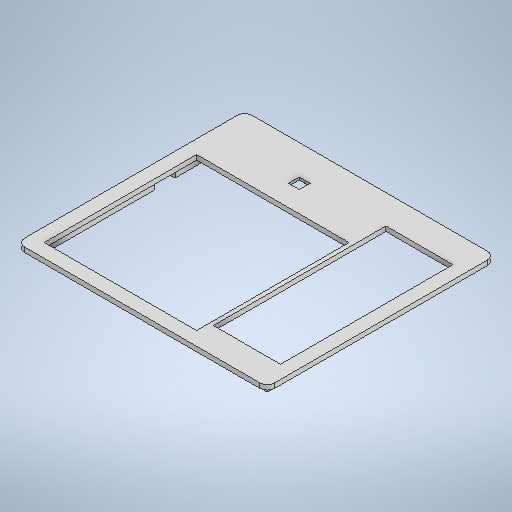
# Autodesk Inventor part: EnclosureLid
Saved by Autodesk Inventor 2025.2 (Build 292293000, 293)
## iProperties
Created: 2025-04-29
Part Number: EnclosureLid
Material: Generic
Document SubType Name: Modeling
Designer: mathe
Density: 1 g/cm^3
Appearance: Default
Author: mathe
Autodesk Inventor part; units mm, degrees
ref_plane "YZ Plane" through (0, 0, 0) normal (1, 0, 0) x (0, 1, 0)
ref_plane "XZ Plane" through (0, 0, 0) normal (0, 1, 0) x (-1, 0, 0)
ref_plane "XY Plane" through (0, 0, 0) normal (0, 0, 1) x (1, 0, 0)
sketch "Sketch1" plane through (0, 0, 0) normal (0, 1, 0) x (-1, 0, 0)
  circle A0 centre (-103.3712, -13.8328) radius 2.5
  circle A1 centre (-103.3712, -93.8328) radius 2.5
  circle A2 centre (-78.3712, -13.8328) radius 2.5
  circle A3 centre (-78.3712, -93.8328) radius 2.5
  line L0 (-8.8712, -9.8328) -> (-107.3712, -9.8328)
  line L1 (-107.3712, -9.8328) -> (-107.3712, -98.8828)
  line L2 (-107.3712, -98.8828) -> (-8.8712, -98.8828)
  line L3 (-8.8712, -98.8828) -> (-8.8712, -69.8328)
  line L4 (-5.8712, -69.8328) -> (-8.8712, -69.8328)
  line L5 (-5.8712, -57.8328) -> (-5.8712, -69.8328)
  line L6 (-5.8712, -57.8328) -> (-8.8712, -57.8328)
  line L7 (-8.8712, -57.8328) -> (-8.8712, -9.8328)
  line L8 (-8.8712, -57.8328) -> (-6.8712, -57.8328)
  line L9 (-6.8712, -57.8328) -> (-6.8712, -69.8328)
  line L10 (-6.8712, -69.8328) -> (-8.8712, -69.8328)
  line L11 (-8.8712, -69.8328) -> (-8.8712, -98.8828)
  line L12 (-8.8712, -98.8828) -> (-107.3712, -98.8828)
  line L13 (-107.3712, -98.8828) -> (-107.3712, -9.8328)
  line L14 (-107.3712, -9.8328) -> (-8.8712, -9.8328)
  line L15 (-8.8712, -9.8328) -> (-8.8712, -57.8328)
  line L16 (-5.8712, -6.8328) -> (-110.3712, -6.8328)
  line L17 (-110.3712, -6.8328) -> (-110.3712, -101.8828)
  line L18 (-110.3712, -101.8828) -> (-5.8712, -101.8828)
  line L19 (-5.8712, -101.8828) -> (-5.8712, -6.8328)
  line L20 (-103.3712, -93.8328) -> (-78.3712, -93.8328) construction
  line L21 (-78.3712, -93.8328) -> (-78.3712, -13.8328) construction
  line L22 (-78.3712, -13.8328) -> (-103.3712, -13.8328) construction
  line L23 (-103.3712, -13.8328) -> (-103.3712, -93.8328) construction
  line L24 (-90.8712, -93.8328) -> (-90.8712, -13.8328) construction
  line L25 (-103.3712, -53.8328) -> (-78.3712, -53.8328) construction
  line L26 (-76.8712, -89.8328) -> (-104.8712, -89.8328)
  line L27 (-104.8712, -89.8328) -> (-104.8712, -17.8328)
  line L28 (-104.8712, -17.8328) -> (-76.8712, -17.8328)
  line L29 (-76.8712, -17.8328) -> (-76.8712, -89.8328)
  line L30 (-76.8712, -89.8328) -> (-104.8712, -17.8328) construction
  line L31 (-104.8712, -89.8328) -> (-76.8712, -17.8328) construction
  line L32 (-9.0712, -58.0328) -> (-7.0712, -58.0328)
  line L33 (-7.0712, -58.0328) -> (-7.0712, -69.6328)
  line L34 (-7.0712, -69.6328) -> (-9.0712, -69.6328)
  line L35 (-9.0712, -69.6328) -> (-9.0712, -98.6828)
  line L36 (-9.0712, -98.6828) -> (-107.1712, -98.6828)
  line L37 (-107.1712, -98.6828) -> (-107.1712, -10.0328)
  line L38 (-107.1712, -10.0328) -> (-9.0712, -10.0328)
  line L39 (-9.0712, -10.0328) -> (-9.0712, -58.0328)
  line L40 (-10.5712, -59.5328) -> (-8.5712, -59.5328)
  line L41 (-8.5712, -59.5328) -> (-8.5712, -68.1328)
  line L42 (-8.5712, -68.1328) -> (-10.5712, -68.1328)
  line L43 (-10.5712, -68.1328) -> (-10.5712, -97.1828)
  line L44 (-10.5712, -97.1828) -> (-105.6712, -97.1828)
  line L45 (-105.6712, -97.1828) -> (-105.6712, -11.5328)
  line L46 (-105.6712, -11.5328) -> (-10.5712, -11.5328)
  line L47 (-10.5712, -11.5328) -> (-10.5712, -59.5328)
  line L48 (-10.5712, -11.5328) -> (-76.1712, -11.5328)
  line L49 (-76.1712, -11.5328) -> (-76.1712, -77.1328)
  line L50 (-76.1712, -77.1328) -> (-10.5712, -77.1328)
  line L51 (-10.5712, -77.1328) -> (-10.5712, -11.5328)
  line L52 (-11.5712, -76.1328) -> (-75.1712, -76.1328)
  line L53 (-75.1712, -76.1328) -> (-75.1712, -12.5328)
  line L54 (-75.1712, -12.5328) -> (-11.5712, -12.5328)
  line L55 (-11.5712, -12.5328) -> (-11.5712, -76.1328)
  line L56 (-76.1712, -77.1328) -> (-10.5712, -77.1328)
  line L57 (-10.5712, -77.1328) -> (-10.5712, -97.1828)
  line L58 (-10.5712, -97.1828) -> (-76.1712, -97.1828)
  line L59 (-76.1712, -97.1828) -> (-76.1712, -77.1328)
  line L60 (-43.3712, -97.1828) -> (-43.3712, -77.1328) construction
  line L61 (-10.5712, -87.1578) -> (-76.1712, -87.1578) construction
  line L62 (-40.1712, -90.3578) -> (-46.5712, -90.3578)
  line L63 (-46.5712, -90.3578) -> (-46.5712, -83.9578)
  line L64 (-46.5712, -83.9578) -> (-40.1712, -83.9578)
  line L65 (-40.1712, -83.9578) -> (-40.1712, -90.3578)
  line L66 (-40.1712, -90.3578) -> (-46.5712, -83.9578) construction
  line L67 (-46.5712, -90.3578) -> (-40.1712, -83.9578) construction
  line L68 (-41.1212, -89.4078) -> (-45.6212, -89.4078)
  line L69 (-45.6212, -89.4078) -> (-45.6212, -84.9078)
  line L70 (-45.6212, -84.9078) -> (-41.1212, -84.9078)
  line L71 (-41.1212, -84.9078) -> (-41.1212, -89.4078)
  line L72 (-41.1212, -89.4078) -> (-45.6212, -84.9078) construction
  line L73 (-45.6212, -89.4078) -> (-41.1212, -84.9078) construction
  point P0 (0, 0)
  point P1 (-90.8712, -53.8328)
  point P2 (-105.6712, -94.8126)
  point P3 (-105.6712, -92.853)
  point P4 (-105.6712, -14.8126)
  point P5 (-105.6712, -12.853)
  point P6 (-104.351, -11.5328)
  point P7 (-102.3914, -11.5328)
  point P8 (-79.351, -11.5328)
  point P9 (-77.3914, -11.5328)
  point P10 (-43.3712, -87.1578)
  dimension "d0" = 28
  dimension "d1" = 72
  dimension "d2" = 0.2
  dimension "d3" = 1.5
  dimension "d10" = 65.6
  dimension "d11" = 65.6
  dimension "d12" = 1
  dimension "d15" = 6.4
  dimension "d16" = 6.4
  dimension "d17" = 4.5
  dimension "d18" = 4.5
  constraints: 148 end point, 16 midpoint, 14 parallel, 7 perpendicular, 6 horizontal, 4 centre point, 17 other
  measures "d0" distance of L27.end L28.end
  measures "d1" distance of L26.end L27.end
  measures "d2" distance between parallel lines of L15 L39
  measures "d3" distance between parallel lines of L39 L47
  measures "d10" distance of L50.end L49.end
  measures "d11" distance of L49.end L48.end
  measures "d12" distance between parallel lines of L50 L52
  measures "d15" distance of L63.end L64.end
  measures "d16" distance of L62.end L63.end
  measures "d17" distance of L69.end L70.end
  measures "d18" distance of L68.end L69.end
extrude "Extrusion1" add sketch "Sketch1" against normal blind 3 contours L46 A0 | A0 L45 | A2 L46 | L45 A1 | L32 L33 L34 L35 L36 L37 L38 L39 picked at (-105.721, -93.6661)
extrude "Extrusion2" add sketch "Sketch1" along normal blind 2 contours A0 L45 L46 | A0 L46 A2 L49 L59 A3 L44 L45 A1 | L46 A0 | A0 L45 | A0 L45 L46 | L46 A2 L49 | A2 L46 | L45 A1 | A1 L45 | L46 L49 A2 | L49 A2 | A2 L49 L46 L47 L51 L43 L50 | L50 L43 L44 L59 A3 | L59 A3 | A3 L59 | L40 L41 L42 L51 | L7 L6 L9 L4 L3 L2 L1 L0 | L0 L1 L2 L3 L4 L19 L18 L17 L16 L6 L7 | L6 L5 L4 L9 | L26 L27 L28 L29 | L32 L33 L34 L35 L36 L37 L38 L39 | L52 L53 L54 L55 | L62 L63 L64 L65 | L68 L69 L70 L71
extrude "Extrusion3" cut sketch "Sketch1" along normal up to surface (2 mm away) contours L26 L27 L28 L29
extrude "Extrusion4" cut sketch "Sketch1" along normal up to surface (2 mm away) contours L52 L53 L54 L55
extrude "Extrusion5" cut sketch "Sketch1" along normal up to surface (2 mm away) contours L68 L69 L70 L71
extrude "Extrusion6" cut sketch "Sketch1" along normal blind 1 contours L62 L63 L64 L65
fillet "Fillet1" radius 3.175 4 edges at (5.8712, 1, -101.8828) (5.8712, 1, -6.8328) (110.3712, 1, -6.8328) (110.3712, 1, -101.8828)
body "Solid1"
